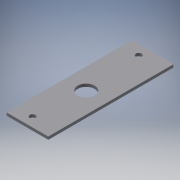
# Autodesk Inventor part: pcb_base
Saved by Autodesk Inventor 2018 (Build 220112000, 112)
## iProperties
Created: 2018-04-04
Part Number: pcb_base
Material: アルミニウム 6061
Document SubType Name: Modeling
Designer: NaMACHAN
Density: 2.7 g/cm^3
Appearance: アルミニウム - フラット
Author: NaMACHAN
Autodesk Inventor part; units mm, degrees
ref_plane "YZ Plane" through (0, 0, 0) normal (1, 0, 0) x (0, 1, 0)
ref_plane "XZ Plane" through (0, 0, 0) normal (0, 1, 0) x (-1, 0, 0)
ref_plane "XY Plane" through (0, 0, 0) normal (0, 0, 1) x (1, 0, 0)
sketch "スケッチ1" plane through (0, 0, 0) normal (0, 0, 1) x (1, 0, 0)
  line L0 (11, -32) -> (-11, -32)
  line L1 (-11, -32) -> (-11, 32)
  line L2 (-11, 32) -> (11, 32)
  line L3 (11, 32) -> (11, -32)
  line L4 (11, -32) -> (-11, 32) construction
  line L5 (-11, -32) -> (11, 32) construction
  point P0 (0, 0)
  dimension "d0" = 22
  dimension "d1" = 64
  constraints: 12 end point, 2 midpoint, 2 parallel, 1 horizontal, 1 perpendicular
  measures "d0" distance of L1.end L2.end
  measures "d1" distance of L0.end L1.end
extrude "押し出し1" add sketch "スケッチ1" along normal blind 1.5
sketch "スケッチ2" plane through (0, 0, 1.5) normal (0, 0, 1) x (1, 0, 0)
  line L0 (-11, 32) -> (-11, -32) projected
  line L1 (11, 32) -> (-11, 32) projected
  line L2 (-11, -32) -> (11, -32) projected
  point P0 (0, 0)
  point P1 (-2.3, 27)
  point P2 (-2.3, -27)
  dimension "d4" = 8.7
  dimension "d5" = 5
  dimension "d6" = 5
  constraints: 1 vertical alignment
  measures "d4" distance from line of L0 point (-2.3, 27)
  measures "d5" distance from line of L1 point (-2.3, 27)
  measures "d6" distance from line of L2 point (-2.3, -27)
hole "穴1" at (-2.3, 27, 1.5) at (-2.3, -27, 1.5) direction (0, 0, -1) diameter 3 end through all
sketch "スケッチ3" plane through (0, 0, 1.5) normal (0, 0, 1) x (1, 0, 0)
  circle A0 centre (0, -3) radius 4.5
  line L0 (11, 32) -> (-11, 32) projected
  point P0 (0, 0)
  dimension "d14" = 35
  dimension "d15" = 9
  constraints: 1 centre point, 1 vertical alignment
  measures "d14" distance from line of L0 A0.centre
  measures "d15" diameter of A0
extrude "押し出し2" cut sketch "スケッチ3" against normal blind 1.5
